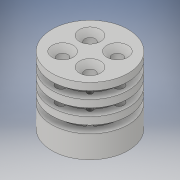
# Autodesk Inventor part: Koło
Saved by Autodesk Inventor 2019 (Build 230136000, 136)
## iProperties
Created: 2021-11-20
Part Number: Koło
Material: Ogólny
Document SubType Name: Modeling
Designer: Michał
Density: 1 g/cm^3
Appearance: Domyślna
Author: Michał
Autodesk Inventor part; units mm, degrees
ref_plane "YZ Plane" through (0, 0, 0) normal (1, 0, 0) x (0, 1, 0)
sketch "Szkic1" plane through (0, 0, 0) normal (0, 1, 0) x (-1, 0, 0)
  circle A0 centre (0, 0) radius 12.5
  circle A1 centre (0, 0) radius 10
  dimension "d0" = 20
  dimension "d2" = 25
  constraints: 2 centre point, 2 coincident
  measures "d0" diameter of A1
  measures "d2" diameter of A0
extrude "Wyciągnięcie proste1" add sketch "Szkic1" along normal blind 5
ref_plane "Płaszczyzna konstrukcyjna1" through (0, -12, 0) normal (0, 0, -1) x (-1, 0, 0)
sketch "Szkic5" plane through (0, -12, 0) normal (0, 0, -1) x (-1, 0, 0)
  line L0 (12.5, 17) -> (-12.5, 17) projected
  line L1 (0, 17) -> (-12.5, 17)
  line L2 (-12.5, 17) -> (-12.5, 19.375)
  line L3 (-12.5, 19.375) -> (0, 19.375)
  line L4 (0, 19.375) -> (0, 17)
  line L5 (0, 19.375) -> (-9.5, 19.375)
  line L6 (-9.5, 19.375) -> (-9.5, 21.875)
  line L7 (-9.5, 21.875) -> (0, 21.875)
  line L8 (0, 21.875) -> (0, 19.375)
  line L9 (0, 21.875) -> (-12.5, 21.875)
  line L10 (-12.5, 21.875) -> (-12.5, 24.25)
  line L11 (-12.5, 24.25) -> (0, 24.25)
  line L12 (0, 24.25) -> (0, 21.875)
  line L13 (0, 24.25) -> (-9.5, 24.25)
  line L14 (-9.5, 24.25) -> (-9.5, 26.75)
  line L15 (-9.5, 26.75) -> (0, 26.75)
  line L16 (0, 26.75) -> (0, 24.25)
  line L17 (0, 26.75) -> (-12.5, 26.75)
  line L18 (-12.5, 26.75) -> (-12.5, 29.125)
  line L19 (-12.5, 29.125) -> (0, 29.125)
  line L20 (0, 29.125) -> (0, 26.75)
  line L21 (0, 29.125) -> (-9.5, 29.125)
  line L22 (-9.5, 29.125) -> (-9.5, 31.625)
  line L23 (-9.5, 31.625) -> (0, 31.625)
  line L24 (0, 31.625) -> (0, 29.125)
  line L25 (0, 31.625) -> (-12.5, 31.625)
  line L26 (-12.5, 31.625) -> (-12.5, 34)
  line L27 (-12.5, 34) -> (0, 34)
  line L28 (0, 34) -> (0, 31.625)
  line L29 (-12.5, 12) -> (-12.5, 17) construction
  line L30 (-12.5, 12) -> (-12.5, 17) construction
  line L31 (-12.5, 12) -> (12.5, 12) construction
  point P0 (0, 12)
  dimension "d13" = 2.5
  dimension "d17" = 22
  dimension "d18" = 3
  constraints: 58 end point, 15 equal length, 7 horizontal, 7 perpendicular, 6 point on line, 5 collinear, 1 midpoint
  measures "d13" distance of L5.end L6.end
  measures "d17" distance between parallel lines of L27 L31
  measures "d18" distance between parallel lines of L26 L22
revolve "Obrót1" add sketch "Szkic5" angle 360 about axis through (0, 12.25, 0) along (0, -1, 0)
sketch "Szkic7" plane through (0, 19.625, 0) normal (0, -1, 0) x (1, 0, 0)
  circle A0 centre (0, 0) radius 9.5 projected
  circle A1 centre (0, 9.5) radius 1.65
  circle A2 centre (0, 0) radius 10 projected
  circle A3 centre (0, 0) radius 9.5 projected
  circle A4 centre (-9.5, 0) radius 1.65
  circle A5 centre (0, -9.5) radius 1.65
  circle A6 centre (9.5, 0) radius 1.65
  circle A7 centre (6.7175, -6.7175) radius 0.9
  circle A8 centre (6.7175, 6.7175) radius 0.9
  circle A9 centre (-6.7175, 6.7175) radius 0.9
  circle A10 centre (-6.7175, -6.7175) radius 0.9
  line L0 (6.7175, 6.7175) -> (0, 0) construction
  line L1 (0, 0) -> (-6.7175, 6.7175) construction
  circle A11 centre (0, 0) radius 12.5 construction
  line L2 (0, 0) -> (-6.7175, -6.7175) construction
  line L3 (0, 0) -> (6.7175, -6.7175) construction
  line L4 (17.5, 0) -> (-17.5, 0) construction
  dimension "d23" = 45
  dimension "d24" = 45
  dimension "d25" = 3.3
  dimension "d47" = 1.8
  constraints: 8 centre point, 8 end point, 8 point on circle, 6 equal radius, 2 collinear
  measures "d23" angle of L4 L1
  measures "d24" angle of L0 L4
  measures "d25" diameter of A1
  measures "d47" diameter of A9
extrude "Wyciągnięcie proste6" cut sketch "Szkic7" along normal up to surface (12.25 mm away) contours A0 A6 | A0 A6 A2 | A8 A0 | A0 A8 A2 | A6 A2 | A7 A2 A0 | A0 A7 | A2 A8 | A7 A2 | A1 A0 | A0 A1 A2 | A5 A2 A0 | A0 A5 | A2 A1 | A5 A2 | A9 A0 | A0 A9 A2 | A10 A2 A0 | A0 A10 | A2 A9 | A10 A2 | A4 A0 | A0 A4 A2 | A2 A4
sketch "Szkic8" plane through (0, -12, 0) normal (0, 0, -1) x (-1, 0, 0)
  line L0 (-1.65, 24.25) -> (1.65, 24.25) projected
  line L1 (-1.65, 29.125) -> (-1.65, 21.875) projected
  line L2 (1.65, 24.25) -> (-1.65, 24.25)
  line L3 (-1.65, 24.25) -> (-1.65, 26.751)
  line L4 (-1.65, 26.751) -> (1.65, 26.751)
  line L5 (1.65, 26.751) -> (1.65, 24.25)
  point P0 (0, 12)
  point P1 (-1.6438, 24.25)
  point P2 (1.6438, 24.25)
  constraints: 8 end point, 2 parallel, 1 horizontal, 1 perpendicular, 1 point on line
extrude "Wyciągnięcie proste7" cut sketch "Szkic8" along normal through all both and the other way through all
sketch "Szkic9" plane through (0, 5, 0) normal (0, -1, 0) x (1, 0, 0)
  line L0 (0, 0) -> (-3.4352, 0)
  line L1 (-3.4352, 0) -> (-3.4352, -2.2657)
  line L2 (-3.4352, -2.2657) -> (0, -2.2657)
  line L3 (0, -2.2657) -> (0, 0)
  dimension "d30" = 3.4352
  dimension "d31" = 2.2658
  constraints: 8 end point, 2 parallel, 1 horizontal, 1 perpendicular
  measures "d30" distance of L1.end L2.end
  measures "d31" distance of L0.end L1.end
extrude "Wyciągnięcie proste8" add sketch "Szkic9" along normal blind 15
ref_plane "Płaszczyzna konstrukcyjna2" through (0, -10, -2.2657) normal (1, 0, 0) x (0, 0, -1)
sketch "Szkic10" plane through (0, -10, 0) normal (0, -1, 0) x (1, 0, 0)
  line L0 (0, 0) -> (-3.4352, 0) projected
  line L1 (-3.4352, -2.2657) -> (0, -2.2657) projected
  line L2 (0, 0) -> (-3.4352, 0)
  line L3 (-3.4352, 0) -> (-3.4352, -2.2657)
  line L4 (-3.4352, -2.2657) -> (0, -2.2657)
  line L5 (0, -2.2657) -> (0, 0)
  constraints: 8 end point, 2 parallel, 1 horizontal, 1 perpendicular
extrude "Wyciągnięcie proste9" cut sketch "Szkic10" against normal up to surface (15 mm away)
sketch "Szkic11" plane through (0, -10, -2.2657) normal (1, 0, 0) x (0, 0, -1)
  line L0 (-3.9095, 22.25) -> (-3.9095, 24.75) projected
  line L1 (-0.622, 22.25) -> (-0.622, 24.75) projected
  line L2 (-3.9095, 22.25) -> (-0.622, 22.25)
  line L3 (-0.622, 22.25) -> (-0.622, 24.75)
  line L4 (-0.622, 24.75) -> (-3.9095, 24.75)
  line L5 (-3.9095, 24.75) -> (-3.9095, 22.25)
  point P0 (-2.2657, 10)
  constraints: 8 end point, 2 parallel, 1 horizontal, 1 perpendicular
extrude "Wyciągnięcie proste10" cut sketch "Szkic11" along normal through all both and the other way through all
sketch "Szkic12" plane through (0, 22, 0) normal (0, 1, 0) x (1, 0, 0)
  line L0 (0, 0) -> (-4.4901, 4.4901) construction
  line L1 (0, 0) -> (0, 6.35) construction
  line L2 (0, 0) -> (-4.4901, -4.4901) construction
  line L3 (0, 0) -> (4.4901, -4.4901) construction
  line L4 (0, 0) -> (4.4901, 4.4901) construction
  circle A0 centre (0, 0) radius 6.35 construction
  circle A1 centre (0, 0) radius 12.5 construction
  point P0 (-4.4901, -4.4901)
  dimension "d48" = 45
  dimension "d49" = 12.7
  constraints: 10 end point, 6 coincident, 4 equal length, 2 collinear, 2 point on circle, 1 centre point, 1 concentric, 1 perpendicular, 1 point on line, 1 vertical
  measures "d48" angle of L4 L1
  measures "d49" diameter of A0
hole "Otwór1" at (-4.4901, 22, -4.4901) at (-4.4901, 22, 4.4901) at (4.4901, 22, 4.4901) at (4.4901, 22, -4.4901) direction (0, -1, 0) diameter 3.4 end through all countersink diameter 6.9 countersink angle 89.954 clearance for "Śruba ze łbem stożkowym ISO 2009/7046" size "M3" standard "ISO"
